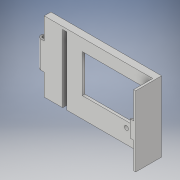
# Autodesk Inventor part: case top_new
Saved by Autodesk Inventor 2017 (Build 210142000, 142)
## iProperties
Created: 2016-12-08
Part Number: case top_new
Material: Generic
Document SubType Name: Modeling
Designer: radrajith
Density: 1 g/cm^3
Appearance: Default
Author: radrajith
Autodesk Inventor part; units mm, degrees
ref_plane "YZ Plane" through (0, 0, 0) normal (1, 0, 0) x (0, 1, 0)
ref_plane "XZ Plane" through (0, 0, 0) normal (0, 1, 0) x (-1, 0, 0)
ref_plane "XY Plane" through (0, 0, 0) normal (0, 0, 1) x (1, 0, 0)
sketch "Sketch1" plane through (0, 0, 0) normal (0, 0, 1) x (1, 0, 0)
  line L0 (0, 0) -> (138.5, 0)
  line L1 (138.5, 0) -> (138.5, 83)
  line L2 (138.5, 83) -> (0, 83)
  line L3 (0, 83) -> (0, 0)
  dimension "d0" = 138.5
  dimension "d1" = 83
  constraints: 8 end point, 2 parallel, 1 horizontal, 1 perpendicular
  measures "d0" distance of L2.end L1.end
  measures "d1" distance of L1.end L0.end
extrude "Extrusion1" add sketch "Sketch1" along normal blind 8
sketch "Sketch2" plane through (0, 0, 8) normal (0, 0, 1) x (1, 0, 0)
  line L0 (138.5, 0) -> (138.5, 83) projected
  line L1 (0, 0) -> (138.5, 0) projected
  line L2 (138.5, 83) -> (136, 83)
  line L3 (136, 83) -> (136, 0)
  line L4 (136, 0) -> (138.5, 0)
  line L5 (138.5, 0) -> (138.5, 83)
  line L6 (0, 83) -> (0, 0) projected
  dimension "d15" = 136
  constraints: 8 end point, 2 parallel, 1 horizontal, 1 perpendicular, 1 point on line
  measures "d15" distance between parallel lines of L3 L6
extrude "Extrusion2" add sketch "Sketch2" along normal blind 22.5
sketch "Sketch3" plane through (136, 0, 8) normal (-1, 0, 0) x (0, 0, 1)
  line L0 (22.5, 0) -> (22.5, 83) projected
  line L1 (22.5, 31.3) -> (20.7, 31.3)
  line L2 (20.7, 31.3) -> (20.7, 51)
  line L3 (20.7, 51) -> (22.5, 51)
  line L4 (22.5, 51) -> (22.5, 31.3)
  point P0 (-8, 0)
  dimension "d6" = 1.8
  constraints: 8 end point, 2 parallel, 1 horizontal, 1 perpendicular, 1 point on line
  measures "d6" distance of L2.end L3.end
extrude "Extrusion3" add sketch "Sketch3" along normal blind 4
sketch "Sketch5" plane through (0, 0, 8) normal (0, 0, 1) x (1, 0, 0)
  line L0 (0, 0) -> (138.5, 0) projected
  line L1 (0, 0) -> (8, 0)
  line L2 (8, 0) -> (8, 25.5)
  line L3 (8, 25.5) -> (0, 25.5)
  line L4 (0, 25.5) -> (0, 0)
  line L5 (0, 83) -> (0, 0) projected
  line L6 (0, 83) -> (8, 83)
  line L7 (8, 83) -> (8, 57.5)
  line L8 (8, 57.5) -> (0, 57.5)
  line L9 (0, 57.5) -> (0, 83)
  dimension "d9" = 8
  dimension "d10" = 25.5
  dimension "d11" = 8
  dimension "d12" = 25.5
  constraints: 16 end point, 4 parallel, 2 horizontal, 2 perpendicular
  measures "d9" distance of L3.end L2.end
  measures "d10" distance of L2.end L1.end
  measures "d11" distance of L7.end L8.end
  measures "d12" distance of L6.end L7.end
extrude "Extrusion4" cut sketch "Sketch5" against normal blind 8
sketch "Sketch6" plane through (0, 25.5, 8) normal (0, -1, 0) x (1, 0, 0)
  circle A0 centre (4, -4) radius 2
  point P0 (0, -8)
  constraints: 1 centre point
extrude "Extrusion5" cut sketch "Sketch6" against normal blind 40
fillet "Fillet1" radius 4 2 edges at (0, 41.5, 8) (0, 41.5, 0)
sketch "Sketch7" plane through (0, 0, 0) normal (0, 0, -1) x (-1, 0, 0)
  line L0 (-115, 24) -> (-53, 24)
  line L1 (-53, 24) -> (-53, 69)
  line L2 (-53, 69) -> (-115, 69)
  line L3 (-115, 69) -> (-115, 24)
  line L4 (-8, 57.5) -> (-8, 83) projected
  line L5 (-138.5, 83) -> (-8, 83) projected
  point P0 (0, 0)
  dimension "d19" = 62
  dimension "d20" = 45
  dimension "d21" = 45
  dimension "d22" = 14
  constraints: 8 end point, 2 parallel, 1 horizontal, 1 perpendicular
  measures "d19" distance of L2.end L1.end
  measures "d20" distance of L1.end L0.end
  measures "d21" distance between parallel lines of L4 L1
  measures "d22" distance between parallel lines of L2 L5
extrude "Extrusion6" cut sketch "Sketch7" against normal blind 10
chamfer "Chamfer1" distance 5 angle 45 4 edges at (115, 46.5, 0) (84, 69, 0) (53, 46.5, 0) (84, 24, 0)
sketch "Sketch8" plane through (0, 0, 8) normal (0, 0, 1) x (1, 0, 0)
  line L0 (115, 69) -> (115, 24) projected
  line L1 (115, 69) -> (125, 69)
  line L2 (125, 69) -> (125, 24)
  line L3 (125, 24) -> (115, 24)
  line L4 (115, 24) -> (115, 69)
  point P0 (0, 0)
  dimension "d28" = 10
  constraints: 8 end point, 2 parallel, 1 horizontal, 1 perpendicular
  measures "d28" distance of L2.end L3.end
extrude "Extrusion7" cut sketch "Sketch8" against normal blind 5
sketch "Sketch9" plane through (0, 0, 8) normal (0, 0, 1) x (1, 0, 0)
  line L0 (8, 0) -> (138.5, 0) projected
  line L1 (34.5, 0) -> (29.7, 0)
  line L2 (29.7, 0) -> (29.7, 80)
  line L3 (29.7, 80) -> (34.5, 80)
  line L4 (34.5, 80) -> (34.5, 0)
  point P0 (0, 0)
  dimension "d31" = 4.8
  constraints: 8 end point, 2 parallel, 1 horizontal, 1 perpendicular, 1 point on line
  measures "d31" distance of L2.end L3.end
extrude "Extrusion8" cut sketch "Sketch9" against normal blind 5
sketch "Sketch10" plane through (0, 0, 8) normal (0, 0, 1) x (1, 0, 0)
  line L0 (29.7, 0) -> (29.7, 80) projected
  line L1 (34.5, 0) -> (29.7, 0)
  line L2 (29.7, 0) -> (29.7, 10)
  line L3 (29.7, 10) -> (34.5, 10)
  line L4 (34.5, 10) -> (34.5, 0)
  point P0 (0, 0)
  constraints: 8 end point, 2 parallel, 1 horizontal, 1 perpendicular, 1 point on line
extrude "Extrusion9" cut sketch "Sketch10" against normal blind 7.2
sketch "Sketch11" plane through (0, 0, 0) normal (0, 0, -1) x (-1, 0, 0)
  circle A0 centre (-105, 17) radius 2.5
  circle A1 centre (-105, 17) radius 2.5
  point P0 (0, 0)
  dimension "d36" = 5
  constraints: 2 centre point, 1 coincident
  measures "d36" diameter of A1
extrude "Extrusion10" cut sketch "Sketch11" against normal blind 8
body "Solid1"
